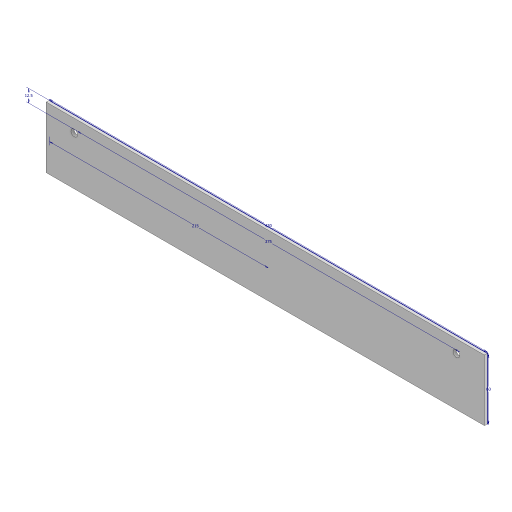
# Autodesk Inventor part: light-trap-panel-bottom-front
Saved by Autodesk Inventor 2023 (Build 270158000, 158)
## iProperties
Created: 2024-07-05
Part Number: light-trap-panel-bottom-front
Material: Generic
Document SubType Name: Modeling
Designer: N.Vladimirov
Density: 1 g/cm^3
Appearance: Default
Author: N.Vladimirov
Autodesk Inventor part; units mm, degrees
ref_plane "YZ Plane" through (0, 0, 0) normal (1, 0, 0) x (0, 1, 0)
ref_plane "XZ Plane" through (0, 0, 0) normal (0, 1, 0) x (-1, 0, 0)
ref_plane "XY Plane" through (0, 0, 0) normal (0, 0, 1) x (1, 0, 0)
sketch "Sketch1" plane through (0, 0, 0) normal (0, 0, 1) x (1, 0, 0)
  line L0 (0, 0) -> (430, 0)
  line L1 (430, 0) -> (430, 60)
  line L2 (430, 60) -> (0, 60)
  line L3 (0, 60) -> (0, 0)
  line L4 (215, 44.8722) -> (215, 13.4403) construction
  point P0 (27.5, 47.5)
  point P1 (402.5, 47.5)
  point P2 (0, 30)
  dimension "d0" = 430
  dimension "d1" = 60
  dimension "d4" = 375
  dimension "d9" = 215
  dimension "d10" = 12.5
  constraints: 10 end point, 2 horizontal, 2 parallel, 1 midpoint, 1 perpendicular, 1 symmetric about line, 1 vertical, 1 other
  measures "d0" distance of L2.end L1.end
  measures "d1" distance of L1.end L0.end
  measures "d4" distance of point (27.5, 47.5) point (402.5, 47.5)
  measures "d9" distance from line of L4 point (0, 30)
  measures "d10" distance from line of point (27.5, 47.5) L2
extrude "Extrusion1" add sketch "Sketch1" along normal blind 3
hole "Hole1" at (27.5, 47.5, 0) at (402.5, 47.5, 0) direction (0, 0, 1) diameter 6.6 end through all clearance for "Flat Head Machine Screw" size "M6" standard "Ansi Metric M Profile"
body "Solid1"
